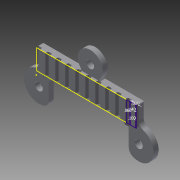
# Autodesk Inventor part: bumpyteethwith3holes
Saved by Autodesk Inventor 2013 SP2 (Build 170200200, 200)
## iProperties
Created: 2015-11-30
Part Number: bumpyteethwith3holes
Document SubType Name: Modeling
Designer: 2016ahoganso
Density: 1 g/cm^3
Material: Generic
Author: 2016ahoganso
Autodesk Inventor part; units mm, degrees
ref_plane "YZ Plane" through (0, 0, 0) normal (1, 0, 0) x (0, 1, 0)
ref_plane "XZ Plane" through (0, 0, 0) normal (0, 1, 0) x (-1, 0, 0)
ref_plane "XY Plane" through (0, 0, 0) normal (0, 0, 1) x (1, 0, 0)
sketch "Sketch1" plane through (0, 0, 0) normal (0, 0, 1) x (1, 0, 0)
  circle A0 centre (5.08, 17.272) radius 2.032
  arc A1 (11.1789, 13.4752) -> (0, 12.192) centre (5.08, 17.272) ccw
  line L0 (11.9198, 12.192) -> (38.8802, 12.192)
  circle A2 centre (45.72, 17.272) radius 2.032
  arc A3 (50.8, 12.192) -> (39.6211, 13.4752) centre (45.72, 17.272) ccw
  line L1 (0, 12.192) -> (0, 2.032)
  line L2 (50.8, 12.192) -> (50.8, 2.032)
  line L3 (11.9198, 12.192) -> (12.7, 12.192)
  line L4 (11.1789, 13.4752) -> (11.9198, 12.192)
  line L5 (38.8802, 12.192) -> (39.6211, 13.4752)
  line L6 (5.1468, 2.032) -> (43.2468, 2.032)
  circle A4 centre (0, -5.588) radius 2.032
  circle A5 centre (50.8, -5.588) radius 2.032
  arc A6 (0, 2.032) -> (7.2193, -8.0264) centre (0, -5.588) ccw
  arc A7 (43.5807, -8.0264) -> (50.8, 2.032) centre (50.8, -5.588) ccw
  line L7 (7.5532, 2.032) -> (7.5532, -7.7724)
  line L8 (7.5532, -7.7724) -> (7.2193, -8.0264)
  line L9 (43.2468, 2.032) -> (44.2342, 2.032)
  line L10 (43.2468, 2.032) -> (43.2468, -7.7724)
  line L11 (43.2468, -7.7724) -> (43.5807, -8.0264)
  line L12 (0, 2.032) -> (0, -5.588)
  line L13 (50.8, 2.032) -> (50.8, -5.588)
  point P0 (10.16, 12.192)
  point P1 (10.16, 2.032)
  dimension "d28" = 11.9198
  dimension "d29" = 4.064
  dimension "d30" = 10.16
  dimension "d31" = 50.8
  dimension "d100" = 38.1
  dimension "d125" = 7.62
  dimension "d126" = 7.62
  constraints: 29 end point, 8 centre point, 8 point on circle, 4 coincident, 3 point on line, 2 parallel, 2 other
  measures "d28" distance of L0.start L1.start
  measures "d29" diameter of A0
  measures "d30" distance between parallel lines of L0 L6
  measures "d31" distance between parallel lines of L2 L1
  measures "d100" distance of L6.start L6.end
  measures "d125" distance of L1.end L12.end
  measures "d126" distance of L2.end L13.end
extrude "Extrusion1" add sketch "Sketch1" along normal blind 6.35
fillet "Fillet5" radius 3.175 2 edges at (50.8, 12.192, 3.175) (50.8, 2.032, 3.175)
fillet "Fillet6" radius 3.175 2 edges at (0, 12.192, 3.175) (0, 2.032, 3.175)
sketch "Sketch2" plane through (0, 0, 6.35) normal (0, 0, 1) x (1, 0, 0)
  line L0 (11.9198, 12.192) -> (38.8802, 12.192) projected
  line L1 (43.2468, 2.032) -> (7.5532, 2.032) projected
  line L2 (0, 2.032) -> (50.8, 2.032)
  line L3 (50.8, 2.032) -> (50.8, 12.192)
  line L4 (50.8, 12.192) -> (0, 12.192)
  line L5 (0, 12.192) -> (0, 2.032)
  line L6 (0, 2.032) -> (2.54, 2.032)
  line L7 (2.54, 12.192) -> (0, 12.192)
  line L8 (0, 12.192) -> (0, 2.032)
  line L9 (2.54, 12.192) -> (5.08, 12.192)
  line L10 (5.08, 2.032) -> (2.54, 2.032)
  line L11 (5.08, 12.192) -> (7.62, 12.192)
  line L12 (7.62, 2.032) -> (5.08, 2.032)
  line L13 (7.62, 12.192) -> (10.16, 12.192)
  line L14 (10.16, 2.032) -> (7.62, 2.032)
  line L15 (10.16, 12.192) -> (12.7, 12.192)
  line L16 (12.7, 2.032) -> (10.16, 2.032)
  line L17 (12.7, 12.192) -> (15.24, 12.192)
  line L18 (15.24, 2.032) -> (12.7, 2.032)
  line L19 (15.2625, 12.192) -> (17.8025, 12.192)
  line L20 (17.8025, 2.032) -> (15.2625, 2.032)
  line L21 (17.8025, 12.192) -> (20.3425, 12.192)
  line L22 (20.3425, 2.032) -> (17.8025, 2.032)
  line L23 (20.3425, 12.192) -> (22.8825, 12.192)
  line L24 (22.8825, 2.032) -> (20.3425, 2.032)
  line L25 (22.8825, 12.192) -> (25.4225, 12.192)
  line L26 (25.4225, 2.032) -> (22.8825, 2.032)
  line L27 (25.4225, 12.192) -> (27.9625, 12.192)
  line L28 (27.9625, 2.032) -> (25.4225, 2.032)
  line L29 (27.9625, 12.192) -> (30.5025, 12.192)
  line L30 (30.5025, 2.032) -> (27.9625, 2.032)
  line L31 (30.5025, 12.192) -> (33.0425, 12.192)
  line L32 (33.0425, 2.032) -> (30.5025, 2.032)
  line L33 (33.0425, 12.192) -> (35.5825, 12.192)
  line L34 (35.5825, 2.032) -> (33.0425, 2.032)
  line L35 (35.5375, 12.192) -> (38.0775, 12.192)
  line L36 (38.0775, 2.032) -> (35.5375, 2.032)
  line L37 (38.0775, 12.192) -> (40.6175, 12.192)
  line L38 (40.6175, 2.032) -> (38.0775, 2.032)
  line L39 (40.6175, 12.192) -> (43.1575, 12.192)
  line L40 (43.1575, 2.032) -> (40.6175, 2.032)
  line L41 (43.1575, 12.192) -> (45.6975, 12.192)
  line L42 (45.6975, 2.032) -> (43.1575, 2.032)
  line L43 (45.6975, 12.192) -> (48.2375, 12.192)
  line L44 (48.2375, 2.032) -> (45.6975, 2.032)
  line L45 (48.2375, 12.192) -> (50.7775, 12.192)
  line L46 (50.7775, 2.032) -> (48.2375, 2.032)
  line L47 (33.0425, 12.192) -> (35.5825, 12.192)
  line L48 (35.5825, 2.032) -> (33.0425, 2.032)
  line L49 (50.7775, 12.192) -> (50.7775, 2.032)
  line L50 (48.2375, 12.192) -> (50.7775, 12.192)
  line L51 (50.7775, 2.032) -> (48.2375, 2.032)
  line L52 (50.7775, 2.032) -> (50.7775, 12.192)
  line L53 (50.7775, 2.032) -> (50.7775, 12.192)
  line L54 (45.6975, 12.192) -> (48.2375, 12.192)
  line L55 (48.2375, 2.032) -> (45.6975, 2.032)
  line L56 (43.1575, 12.192) -> (45.6975, 12.192)
  line L57 (45.6975, 2.032) -> (43.1575, 2.032)
  line L58 (40.6175, 12.192) -> (43.1575, 12.192)
  line L59 (43.1575, 2.032) -> (40.6175, 2.032)
  line L60 (38.0775, 12.192) -> (40.6175, 12.192)
  line L61 (40.6175, 2.032) -> (38.0775, 2.032)
  line L62 (35.5375, 12.192) -> (38.0775, 12.192)
  line L63 (38.0775, 2.032) -> (35.5375, 2.032)
  point P0 (6.096, 2.032)
  point P1 (44.704, 2.032)
  point P2 (0, 0)
  dimension "d43" = 50.8
  constraints: 124 end point, 29 parallel, 28 horizontal, 4 point on line, 2 perpendicular
  measures "d43" distance of L2.start L2.end
extrude "Extrusion2" add sketch "Sketch2" along normal blind 1.2446
sketch "Sketch3" plane through (0, 0, 7.5946) normal (0, 0, 1) x (1, 0, 0)
  line L0 (0, 2.032) -> (0, 12.192) projected
  line L1 (50.8, 2.032) -> (0, 2.032) projected
  line L2 (50.8, 12.192) -> (50.8, 2.032) projected
  line L3 (0, 12.192) -> (50.8, 12.192) projected
  line L4 (50.8, 12.192) -> (47.244, 12.192)
  line L5 (47.244, 12.192) -> (47.244, 2.032)
  line L6 (47.244, 2.032) -> (50.8, 2.032)
  line L7 (50.8, 2.032) -> (50.8, 12.192)
  line L8 (47.244, 12.192) -> (45.72, 12.192)
  line L9 (45.72, 12.192) -> (45.72, 2.032)
  line L10 (45.72, 2.032) -> (47.244, 2.032)
  line L11 (47.244, 2.032) -> (47.244, 12.192)
  line L12 (50.8, 12.192) -> (50.292, 12.192)
  line L13 (50.292, 12.192) -> (47.752, 12.192)
  line L14 (47.752, 12.192) -> (47.752, 2.032)
  line L15 (47.752, 2.032) -> (50.292, 2.032)
  line L16 (50.292, 2.032) -> (50.292, 12.192)
  point P0 (0, 0)
  dimension "d71" = 3.556
  dimension "d72" = 1.524
  dimension "d73" = 0.508
  dimension "d74" = 2.54
  constraints: 26 end point, 6 parallel, 4 point on line, 3 horizontal, 3 perpendicular
  measures "d71" distance between parallel lines of L5 L7
  measures "d72" distance between parallel lines of L9 L11
  measures "d73" distance of L2.start L12.end
  measures "d74" distance between parallel lines of L14 L16
sketch "Sketch4" plane through (0, 12.192, 6.35) normal (0, 1, 0) x (1, 0, 0)
  line L0 (0, -1.2446) -> (50.8, -1.2446) projected
  line L1 (50.8, 0) -> (50.8, -1.2446) projected
  line L2 (0, 0) -> (50.8, 0) projected
  line L3 (50.8, 0) -> (50.292, 0)
  line L4 (50.292, 0) -> (50.292, -1.2446)
  line L5 (50.292, -1.2446) -> (50.8, 0)
  point P0 (35.5375, 0)
  point P1 (0, 6.35)
  dimension "d75" = 0.508
  constraints: 6 end point, 2 point on line, 1 perpendicular
  measures "d75" distance of L1.start L3.end
extrude "Extrusion3" cut sketch "Sketch4" against normal blind 25.4 contours L5 L1 L0
sketch "Sketch5" plane through (6.096, 2.032, 0) normal (0, -1, 0) x (1, 0, 0)
  line L0 (44.196, 7.5946) -> (-6.096, 7.5946) projected
  line L1 (-6.096, 6.35) -> (-6.096, 7.5946) projected
  line L2 (44.704, 6.35) -> (-6.096, 6.35) projected
  line L3 (44.704, 6.35) -> (41.148, 6.35)
  line L4 (41.656, 7.5946) -> (41.148, 6.35)
  line L5 (41.148, 6.35) -> (39.624, 6.35)
  line L6 (39.624, 6.35) -> (39.116, 7.5946)
  line L7 (44.196, 7.5946) -> (41.656, 7.5946)
  line L8 (36.576, 7.5946) -> (36.068, 6.35)
  line L9 (36.068, 6.35) -> (34.544, 6.35)
  line L10 (34.544, 6.35) -> (34.036, 7.5946)
  line L11 (39.116, 7.5946) -> (36.576, 7.5946)
  line L12 (31.496, 7.5946) -> (30.988, 6.35)
  line L13 (30.988, 6.35) -> (29.464, 6.35)
  line L14 (29.464, 6.35) -> (28.956, 7.5946)
  line L15 (34.036, 7.5946) -> (31.496, 7.5946)
  line L16 (26.416, 7.5946) -> (25.908, 6.35)
  line L17 (25.908, 6.35) -> (24.384, 6.35)
  line L18 (24.384, 6.35) -> (23.876, 7.5946)
  line L19 (28.956, 7.5946) -> (26.416, 7.5946)
  line L20 (21.336, 7.5946) -> (20.828, 6.35)
  line L21 (20.828, 6.35) -> (19.304, 6.35)
  line L22 (19.304, 6.35) -> (18.796, 7.5946)
  line L23 (23.876, 7.5946) -> (21.336, 7.5946)
  line L24 (16.256, 7.5946) -> (15.748, 6.35)
  line L25 (15.748, 6.35) -> (14.224, 6.35)
  line L26 (14.224, 6.35) -> (13.716, 7.5946)
  line L27 (18.796, 7.5946) -> (16.256, 7.5946)
  line L28 (11.176, 7.5946) -> (10.668, 6.35)
  line L29 (10.668, 6.35) -> (9.144, 6.35)
  line L30 (9.144, 6.35) -> (8.636, 7.5946)
  line L31 (13.716, 7.5946) -> (11.176, 7.5946)
  line L32 (6.096, 7.5946) -> (5.588, 6.35)
  line L33 (5.588, 6.35) -> (4.064, 6.35)
  line L34 (4.064, 6.35) -> (3.556, 7.5946)
  line L35 (8.636, 7.5946) -> (6.096, 7.5946)
  line L36 (1.016, 7.5946) -> (0.508, 6.35)
  line L37 (0.508, 6.35) -> (-1.016, 6.35)
  line L38 (-1.016, 6.35) -> (-1.524, 7.5946)
  line L39 (3.556, 7.5946) -> (1.016, 7.5946)
  line L40 (-4.064, 7.5946) -> (-4.572, 6.35)
  line L41 (-4.572, 6.35) -> (-6.096, 6.35)
  line L42 (-1.524, 7.5946) -> (-4.064, 7.5946)
  line L43 (-6.096, 6.35) -> (-6.096, 7.5946)
  line L44 (-4.064, 7.5946) -> (-6.096, 7.5946)
  line L45 (-1.524, 7.5946) -> (1.016, 7.5946)
  line L46 (3.556, 7.5946) -> (6.3889, 7.5946)
  line L47 (8.636, 7.5946) -> (11.6007, 7.5946)
  line L48 (13.716, 7.5946) -> (41.656, 7.5946)
  line L49 (3.556, 7.5946) -> (6.096, 7.5946)
  line L50 (8.636, 7.5946) -> (11.176, 7.5946)
  line L51 (13.716, 7.5946) -> (16.256, 7.5946)
  line L52 (18.796, 7.5946) -> (21.336, 7.5946)
  line L53 (23.876, 7.5946) -> (26.416, 7.5946)
  line L54 (28.956, 7.5946) -> (31.496, 7.5946)
  line L55 (34.036, 7.5946) -> (36.576, 7.5946)
  line L56 (39.116, 7.5946) -> (41.656, 7.5946)
  point P0 (38.608, 6.35)
  point P1 (-6.096, 0)
  dimension "d78" = 3.556
  dimension "d80" = 1.524
  dimension "d82" = 1.524
  dimension "d83" = 1.524
  dimension "d84" = 1.524
  dimension "d85" = 1.524
  dimension "d86" = 1.524
  dimension "d87" = 1.524
  dimension "d88" = 1.524
  dimension "d89" = 1.524
  dimension "d90" = 1.524
  constraints: 108 end point, 12 collinear, 6 point on line, 1 perpendicular
  measures "d78" distance of L2.start L3.end
  measures "d80" distance of L3.end L5.end
  measures "d82" distance of L8.end L9.end
  measures "d83" distance of L12.end L13.end
  measures "d84" distance of L16.end L17.end
  measures "d85" distance of L20.end L21.end
  measures "d86" distance of L24.end L25.end
  measures "d87" distance of L28.end L29.end
  measures "d88" distance of L32.end L33.end
  measures "d89" distance of L36.end L37.end
  measures "d90" distance of L40.end L1.start
extrude "Extrusion4" cut sketch "Sketch5" against normal blind 25.4 contours L4 L2 L6 L0 | L8 L2 L10 L0 | L12 L2 L14 L0 | L16 L2 L18 L0 | L20 L2 L22 L0 | L24 L2 L26 L0 | L28 L2 L30 L0 | L2 L34 L0 L32 | L2 L38 L0 L36 | L2 L1 L0 L40
sketch "Sketch9" plane through (0, 0, 0) normal (0, 0, -1) x (-1, 0, 0)
  line L0 (-38.8802, 12.192) -> (-11.9198, 12.192) projected
  line L1 (-7.2193, -8.0264) -> (-7.5532, -7.7724) projected
  line L2 (-25.4, 12.192) -> (-26.924, 12.192) projected
  line L3 (-26.162, 12.192) -> (-26.162, 17.272)
  line L4 (-26.162, 12.192) -> (-21.082, 12.192) construction
  circle A0 centre (-26.162, 17.272) radius 2.032
  arc A1 (-22.352, 12.192) -> (-29.972, 12.192) centre (-26.162, 17.272) ccw
  line L5 (-22.352, 12.192) -> (-29.972, 12.192)
  line L6 (-21.082, 12.192) -> (-21.6207, 12.8336)
  line L7 (-30.48, 12.192) -> (-32.004, 12.192) projected
  line L8 (-31.242, 12.192) -> (-30.7317, 12.8629)
  line L9 (-21.082, 12.192) -> (-22.352, 12.192)
  point P0 (0, 0)
  dimension "d102" = 5.08
  dimension "d103" = 90
  dimension "d105" = 4.064
  constraints: 12 end point, 4 point on circle, 3 perpendicular, 2 centre point, 2 coincident, 2 collinear, 2 midpoint, 1 horizontal
  measures "d102" distance of L3.start L3.end
  measures "d103" angle of L4 L3
  measures "d105" diameter of A0
extrude "Extrusion6" add sketch "Sketch9" against normal blind 6.35
sketch "Sketch10" plane through (0, 0, 6.35) normal (0, 0, 1) x (1, 0, 0)
  circle A0 centre (45.72, 17.272) radius 2.032 projected
  line L0 (37.592, 12.192) -> (57.4914, 12.192)
  line L1 (57.4914, 12.192) -> (57.4914, 25.728)
  line L2 (57.4914, 25.728) -> (37.592, 25.728)
  line L3 (37.592, 25.728) -> (37.592, 12.192)
  line L4 (21.082, 12.192) -> (11.9198, 12.192) projected
  line L5 (13.7364, 12.192) -> (-3.3231, 12.192)
  line L6 (-3.3231, 12.192) -> (-3.3231, 25.728)
  line L7 (-3.3231, 25.728) -> (13.7364, 25.728)
  line L8 (13.7364, 25.728) -> (13.7364, 12.192)
  point P0 (0, 0)
  constraints: 16 end point, 4 parallel, 2 horizontal, 2 perpendicular, 1 point on line
extrude "Extrusion7" cut sketch "Sketch10" against normal blind 8.4667
sketch "Sketch11" plane through (0, 0, 0) normal (0, 0, -1) x (-1, 0, 0)
  circle A0 centre (0, -5.588) radius 2.032 projected
  circle A1 centre (-50.8, -5.588) radius 2.032 projected
  circle A2 centre (-26.162, 17.272) radius 2.032 projected
  line L0 (0.2268, 12.192) -> (-21.082, 12.192) projected
  line L1 (-21.082, 12.192) -> (-21.6207, 12.8336) projected
  arc A3 (-21.6207, 12.8336) -> (-30.7317, 12.8629) centre (-26.162, 17.272) ccw projected
  line L2 (-30.7317, 12.8629) -> (-31.242, 12.192) projected
  line L3 (-51.0268, 12.192) -> (-31.242, 12.192) projected
  arc A4 (-50.8, 11.0136) -> (-51.0268, 12.192) centre (-53.975, 11.0136) ccw projected
  line L4 (-50.8, 4.7295) -> (-50.8, 11.0136) projected
  arc A5 (-53.0412, 1.695) -> (-50.8, 4.7295) centre (-53.975, 4.7295) ccw projected
  arc A6 (-53.0412, 1.695) -> (-43.5807, -8.0264) centre (-50.8, -5.588) ccw projected
  line L5 (-43.2468, -7.7724) -> (-43.5807, -8.0264) projected
  line L6 (-43.2468, 2.032) -> (-43.2468, -7.7724) projected
  line L7 (-7.5532, 2.032) -> (-43.2468, 2.032) projected
  line L8 (-7.5532, -7.7724) -> (-7.5532, 2.032) projected
  line L9 (-7.2193, -8.0264) -> (-7.5532, -7.7724) projected
  arc A7 (-7.2193, -8.0264) -> (2.2412, 1.695) centre (0, -5.588) ccw projected
  arc A8 (0, 4.7295) -> (2.2412, 1.695) centre (3.175, 4.7295) ccw projected
  line L10 (0, 11.0136) -> (0, 4.7295) projected
  arc A9 (0.2268, 12.192) -> (0, 11.0136) centre (3.175, 11.0136) ccw projected
  point P0 (0, 0)
extrude "Extrusion8" cut sketch "Sketch11" against normal blind 3.81
sketch "Sketch12" plane through (7.5532, -7.7724, 6.35) normal (1, 0, 0) x (0, 0, -1)
  line L0 (2.54, 0) -> (2.54, 9.8044) projected
  line L1 (2.54, 9.8044) -> (0, 9.8044) projected
  line L2 (0, 9.8044) -> (0, 0) projected
  line L3 (2.54, 0) -> (0, 0) projected
  point P0 (6.35, 7.7724)
extrude "Extrusion9" cut sketch "Sketch12" against normal blind 2.54
sketch "Sketch13" plane through (5.0132, -7.7724, 3.81) normal (0, 1, 0) x (1, 0, 0)
  line L0 (2.54, 0) -> (2.54, -2.54) projected
  line L1 (0, 0) -> (2.54, 0) projected
  line L2 (0, 0) -> (0, -2.54) projected
  line L3 (2.54, -2.54) -> (0, -2.54) projected
  point P0 (-5.0132, 3.81)
extrude "Extrusion10" cut sketch "Sketch13" against normal blind 25.4
sketch "Sketch14" plane through (43.2468, -7.7724, 6.35) normal (-1, 0, 0) x (0, 0, 1)
  line L0 (-2.54, 9.8044) -> (-2.54, 0) projected
  line L1 (-2.54, 0) -> (0, 0) projected
  line L2 (0, 0) -> (0, 9.8044) projected
  line L3 (-2.54, 9.8044) -> (0, 9.8044) projected
  point P0 (-6.35, 7.7724)
extrude "Extrusion11" cut sketch "Sketch14" against normal blind 2.54
sketch "Sketch15" plane through (43.2468, -7.7724, 6.35) normal (0, 1, 0) x (1, 0, 0)
  line L0 (0, 2.54) -> (0, 0) projected
  line L1 (2.54, 0) -> (0, 0) projected
  line L2 (2.54, 0) -> (2.54, 2.54) projected
  line L3 (0, 2.54) -> (2.54, 2.54) projected
  point P0 (-43.2468, 6.35)
extrude "Extrusion12" cut sketch "Sketch15" against normal blind 25.4
fillet "Fillet7" radius 3.175 1 edges at (45.7868, -11.3266, 5.08)
fillet "Fillet8" radius 3.175 1 edges at (5.0132, -11.3266, 5.08)
fillet "Fillet9" radius 3.175 1 edges at (5.0132, 2.032, 5.08)
fillet "Fillet10" radius 3.175 1 edges at (45.7868, 2.032, 5.08)
body "Solid1"
